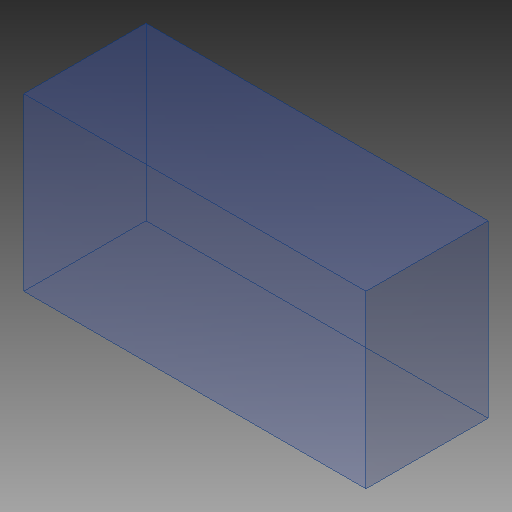
# Autodesk Inventor part: 測定ボックス
Saved by Autodesk Inventor 2020 (Build 240168000, 168)
## iProperties
Part Number: 測定ボックス
Material: 空気
Document SubType Name: Modeling
Designer: 雪村
Appearance: トロピカル 青
Surface Area: 10150 cm^2
Volume: 61250 cm^3
Author: 雪村
Autodesk Inventor part; units mm, degrees
ref_plane "YZ Plane" through (0, 0, 0) normal (1, 0, 0) x (0, 1, 0)
ref_plane "XZ Plane" through (0, 0, 0) normal (0, 1, 0) x (-1, 0, 0)
ref_plane "XY Plane" through (0, 0, 0) normal (0, 0, 1) x (1, 0, 0)
sketch "スケッチ1" plane through (0, 0, 0) normal (0, 0, 1) x (1, 0, 0)
  line L0 (0, 0) -> (700, 0)
  line L1 (700, 0) -> (700, 350)
  line L2 (700, 350) -> (0, 350)
  line L3 (0, 350) -> (0, 0)
  dimension "d0" = 700
  dimension "d1" = 350
  constraints: 8 end point
  measures "d0" distance of L2.end L1.end
  measures "d1" distance of L1.end L0.end
extrude "押し出し1" add sketch "スケッチ1" along normal blind 250
